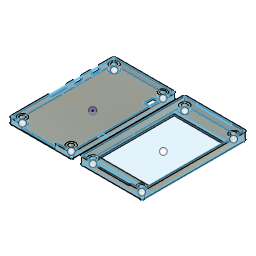
ProjectSpectre (Autodesk Fusion 360 design; units mm, degrees)
Autodesk Fusion 360 part; units mm, degrees
sketch "Sketch1" plane through (0, 0, 0) normal (0, 0, 1) x (1, 0, 0)
  line L0 (-25.25, 0) -> (-25.25, 43.25)
  line L1 (25.25, 0) -> (25.25, 43.25)
  line L2 (-25.25, 0) -> (-25.25, -43.25)
  line L3 (25.25, 0) -> (25.25, -43.25)
  line L4 (-25.25, 43.25) -> (25.25, 43.25)
  line L5 (-25.25, -43.25) -> (25.25, -43.25)
  circle A0 centre (-20.75, 39) radius 2.1
  circle A1 centre (20.75, 39) radius 2.1
  circle A2 centre (-20.75, -39) radius 2.1
  circle A3 centre (20.75, -39) radius 2.1
  line L6 (-25.25, 43.25, 0) -> (-25.25, 43.25, 4.5)
  line L7 (25.25, 43.25, 0) -> (25.25, 43.25, 4.5)
  line L8 (25.25, -43.25, 0) -> (25.25, -43.25, 4.5)
  line L9 (-25.25, -43.25, 0) -> (-25.25, -43.25, 4.5)
  line L10 (25.25, 43.25, 4.5) -> (25.25, -43.25, 4.5)
  line L11 (-25.25, -43.25, 4.5) -> (-25.25, 43.25, 4.5)
  line L12 (-25.25, 43.25, 4.5) -> (25.25, 43.25, 4.5)
  line L13 (-25.25, 43.25, 4.5) -> (-25.25, 31.55, 4.5)
  line L14 (-25.25, 31.55, 4.5) -> (-25.25, 31.55, 1)
  line L15 (-25.25, 31.55, 1) -> (-25.25, 24.55, 1)
  line L16 (-25.25, 24.55, 1) -> (-25.25, 24.55, 4.5)
  line L17 (-25.25, 24.55, 4.5) -> (-25.25, 16.65, 4.5)
  line L18 (-25.25, 16.65, 4.5) -> (-25.25, 16.65, 1)
  line L19 (-25.25, 16.65, 1) -> (-25.25, 9.65, 1)
  line L20 (-25.25, 9.65, 1) -> (-25.25, 9.65, 4.5)
  line L21 (21.95, 35.45) -> (21.95, 27.45)
  line L22 (21.95, 27.45) -> (15.85, 27.45)
  line L23 (15.85, 27.45) -> (15.85, 35.45)
  line L24 (15.85, 35.45) -> (21.95, 35.45)
  line L25 (-25.25, 9.65, 4.5) -> (-25.25, 4, 4.5)
  line L26 (-25.25, 4, 4.5) -> (-25.25, 4, 2.5)
  line L27 (-25.25, 4, 2.5) -> (-25.25, -11, 2.5)
  line L28 (-25.25, -11, 2.5) -> (-25.25, -11, 4.5)
  line L29 (24.25, -16.75) -> (24.25, -12.45)
  line L30 (24.25, -12.45) -> (21.35, -12.45)
  line L31 (21.35, -12.45) -> (21.35, -16.75)
  line L32 (21.35, -16.75) -> (24.25, -16.75)
  circle A4 centre (20.75, -39) radius 3.75
  circle A5 centre (-20.75, -39) radius 3.75
  circle A6 centre (-20.75, 39) radius 3.75
  circle A7 centre (20.75, 39) radius 3.5
  line L33 (-25.25, -43.25, 4.5) -> (-15.75, -43.25, 4.5)
  line L34 (-15.75, -43.25, 4.5) -> (-15.75, -43.25, 1)
  line L35 (-15.75, -43.25, 1) -> (13.05, -43.25, 1)
  line L36 (13.05, -43.25, 1) -> (13.05, -43.25, 4.5)
  line L37 (13.05, -43.25, 4.5) -> (25.25, -43.25, 4.5)
  line L38 (24.25, -12.45) -> (21.35, -12.45)
  line L39 (21.95, 27.45) -> (15.85, 27.45)
  line L40 (-25.25, -43.25, 0) -> (-25.25, -43.25, 4.5)
  line L41 (-25.25, 4, 4.5) -> (-25.25, 4, 2.5)
  line L42 (-25.25, 0) -> (-25.25, -43.25)
  line L43 (-25.25, -43.25, 4.5) -> (-15.75, -43.25, 4.5)
  line L44 (-25.25, 4, 2.5) -> (-25.25, -11, 2.5)
  circle A8 centre (20.75, 39) radius 2.1
  line L45 (-25.25, -43.25) -> (25.25, -43.25)
  line L46 (-25.25, 31.55, 4.5) -> (-25.25, 31.55, 1)
  line L47 (25.25, -43.25, 0) -> (25.25, -43.25, 4.5)
  circle A9 centre (20.75, -39) radius 3.75
  line L48 (15.85, 27.45) -> (15.85, 35.45)
  line L49 (-25.25, 0) -> (-25.25, 43.25)
  line L50 (21.35, -16.75) -> (24.25, -16.75)
  line L51 (-25.25, 43.25, 0) -> (-25.25, 43.25, 4.5)
  line L52 (13.05, -43.25, 4.5) -> (25.25, -43.25, 4.5)
  circle A10 centre (-20.75, 39) radius 2.1
  line L53 (21.35, -12.45) -> (21.35, -16.75)
  circle A11 centre (20.75, 39) radius 3.5
  line L54 (15.85, 35.45) -> (21.95, 35.45)
  line L55 (25.25, 0) -> (25.25, -43.25)
  line L56 (24.25, -16.75) -> (24.25, -12.45)
  line L57 (13.05, -43.25, 1) -> (13.05, -43.25, 4.5)
  circle A12 centre (20.75, -39) radius 2.1
  line L58 (-25.25, 43.25) -> (25.25, 43.25)
  line L59 (21.95, 35.45) -> (21.95, 27.45)
  line L60 (-25.25, 43.25, 4.5) -> (25.25, 43.25, 4.5)
  line L61 (25.25, 43.25, 0) -> (25.25, 43.25, 4.5)
  circle A13 centre (-20.75, 39) radius 3.75
  line L62 (-25.25, -43.25, 4.5) -> (-25.25, 43.25, 4.5)
  line L63 (-25.25, 9.65, 4.5) -> (-25.25, 4, 4.5)
  line L64 (25.25, 0) -> (25.25, 43.25)
  line L65 (25.25, 43.25, 4.5) -> (25.25, -43.25, 4.5)
  line L66 (-25.25, 43.25, 4.5) -> (-25.25, 31.55, 4.5)
  line L67 (-25.25, 31.55, 1) -> (-25.25, 24.55, 1)
  line L68 (-15.75, -43.25, 1) -> (13.05, -43.25, 1)
  line L69 (-25.25, 24.55, 1) -> (-25.25, 24.55, 4.5)
  line L70 (-25.25, 16.65, 4.5) -> (-25.25, 16.65, 1)
  line L71 (-25.25, 16.65, 1) -> (-25.25, 9.65, 1)
  line L72 (-15.75, -43.25, 4.5) -> (-15.75, -43.25, 1)
  line L73 (-25.25, 9.65, 1) -> (-25.25, 9.65, 4.5)
  line L74 (-25.25, -11, 2.5) -> (-25.25, -11, 4.5)
  circle A14 centre (-20.75, -39) radius 3.75
  line L75 (-25.25, 24.55, 4.5) -> (-25.25, 16.65, 4.5)
  circle A15 centre (-20.75, -39) radius 2.1
  dimension "d5" = 41.5
  dimension "d7" = 78
  dimension "d8" = 25.25
  dimension "d9" = 25.25
  dimension "d12" = 43.25
  dimension "d13" = 43.25
  dimension "d14" = 43.25
  dimension "d15" = 43.25
  dimension "d16" = 4.2
  dimension "d17" = 4.2
  dimension "d18" = 4.2
  dimension "d19" = 4.2
  dimension "d28" = 4.5
  dimension "d29" = 4.5
  dimension "d30" = 4.5
  dimension "d31" = 4.5
  dimension "d32" = 11.7
  dimension "d33" = 3.5
  dimension "d34" = 7
  dimension "d35" = 3.5
  dimension "d36" = 7.9
  dimension "d37" = 3.5
  dimension "d38" = 7
  dimension "d39" = 3.5
  dimension "d42" = 8
  dimension "d43" = 6.1
  dimension "d44" = 8
  dimension "d45" = 5.65
  dimension "d46" = 2
  dimension "d47" = 15
  dimension "d54" = 4.3
  dimension "d55" = 2.9
  dimension "d56" = 4.3
  dimension "d57" = 7.5
  dimension "d58" = 7.5
  dimension "d59" = 7.5
  dimension "d60" = 7
  dimension "d62" = 9.5
  dimension "d63" = 3.5
  dimension "d64" = 28.8
  dimension "d65" = 3.5
  dimension "d100" = 41.5
  dimension "d101" = 78
  dimension "d103" = 43.25
  dimension "d104" = 43.25
  dimension "d105" = 43.25
  dimension "d106" = 43.25
  dimension "d107" = 4.2
  dimension "d108" = 4.2
  dimension "d109" = 4.2
  dimension "d110" = 4.2
  dimension "d111" = 4.5
  dimension "d112" = 4.5
  dimension "d113" = 4.5
  dimension "d114" = 4.5
  dimension "d115" = 11.7
  dimension "d116" = 3.5
  dimension "d117" = 7
  dimension "d118" = 3.5
  dimension "d119" = 7.9
  dimension "d120" = 3.5
  dimension "d121" = 7
  dimension "d122" = 3.5
  dimension "d123" = 8
  dimension "d124" = 6.1
  dimension "d125" = 8
  dimension "d126" = 5.65
  dimension "d127" = 2
  dimension "d128" = 15
  dimension "d129" = 4.3
  dimension "d130" = 2.9
  dimension "d131" = 4.3
  dimension "d132" = 7.5
  dimension "d133" = 7.5
  dimension "d134" = 7.5
  dimension "d135" = 7
  dimension "d136" = 9.5
  dimension "d137" = 3.5
  dimension "d138" = 28.8
  dimension "d139" = 3.5
  constraint perpendicular L22 L23
  constraint perpendicular L29 L30
  constraint perpendicular L30 L31
  constraint concentric A3 A4
  constraint concentric A2 A5
  constraint concentric A0 A6
  constraint concentric A1 A7
  constraint perpendicular L39 L48
  constraint perpendicular L38 L56
  constraint perpendicular L38 L53
  constraint concentric A9 A12
  constraint concentric A14 A15
  constraint concentric A10 A13
  constraint concentric A8 A11
  measures "d5" distance of A0.centre A1.centre
  measures "d7" distance of A0.centre A2.centre
  measures "d8" distance of origin L1.start
  measures "d9" distance of origin L0.start
  measures "d12" distance of L0.start L0.end
  measures "d13" distance of L1.start L1.end
  measures "d14" distance of L0.start L2.end
  measures "d15" distance of L1.start L3.end
  measures "d16" diameter of A0
  measures "d17" diameter of A1
  measures "d18" diameter of A2
  measures "d19" diameter of A3
  measures "d28" distance of L0.end L4.start
  measures "d29" distance of L1.end L4.end
  measures "d30" distance of L3.end L5.end
  measures "d31" distance of L2.end L5.start
  measures "d42" distance of L21.start L21.end
  measures "d43" distance of L21.end L22.end
  measures "d44" distance of L22.end L23.end
  measures "d54" distance of L29.start L29.end
  measures "d55" distance of L29.end L30.end
  measures "d56" distance of L30.end L31.end
  measures "d57" diameter of A4
  measures "d58" diameter of A5
  measures "d59" diameter of A6
  measures "d60" diameter of A7
  measures "d100" distance of A1.centre A0.centre
  measures "d101" distance of A2.centre A0.centre
  measures "d103" distance of L0.start L0.end
  measures "d104" distance of L1.end L1.start
  measures "d105" distance of L0.start L2.end
  measures "d106" distance of L3.end L1.start
  measures "d107" diameter of A10
  measures "d108" diameter of A8
  measures "d109" diameter of A15
  measures "d110" diameter of A12
  measures "d111" distance of L0.end L4.start
  measures "d112" distance of L1.end L4.end
  measures "d113" distance of L3.end L5.end
  measures "d114" distance of L2.end L5.start
  measures "d123" distance of L21.start L21.end
  measures "d124" distance of L22.end L21.end
  measures "d125" distance of L22.end L23.end
  measures "d129" distance of L29.start L29.end
  measures "d130" distance of L30.end L29.end
  measures "d131" distance of L31.end L30.end
  measures "d132" diameter of A9
  measures "d133" diameter of A14
  measures "d134" diameter of A13
  measures "d135" diameter of A11
extrude "Extrude1" add sketch "Sketch1" against normal blind 1.5 contours L1 L3 L7 L8 L10 L47 L55 L61 L64 L65 in plane through (25.25, 0, 0) normal (1, 0, 0) makes body 1
extrude "Extrude2" add sketch "Sketch1" along normal blind 1.5 contours L4 L6 L7 L12 L51 L58 L60 L61 in plane through (0, 43.25, 0) normal (0, 1, 0) bodies 1
extrude "Extrude3" add 1 faces at (-25.25, 43.75, 1.5) along direction (-1, 0, 0) blind 1.5 on bodies 1 bodies 1
extrude "Extrude4" add sketch "Sketch1" against normal blind 1.5 contours L0 L2 L6 L9 L11 L13 L14 L15 L16 L17 L18 L19 L20 L25 L26 L27 L28 L40 L41 L42 L44 L46 L49 L51 L62 L63 L66 L67 L69 L70 L71 L73 L74 L75 in plane through (-25.25, 0, 0) normal (1, 0, 0) bodies 1
extrude "Extrude5" cut 1 faces at (23.75, 14.4167, 1.5) along direction (1, 0, 0) blind 3 on bodies 1 bodies 1
extrude "Extrude6" add 1 faces at (25.25, 44.25, 1.5) along direction (1, 0, 0) blind 1.5 on bodies 1 bodies 1
extrude "Extrude7" add sketch "Sketch1" against normal blind 1.5 contours L1 L3 L7 L8 L10 L47 L55 L61 L64 L65 in plane through (25.25, 0, 0) normal (1, 0, 0) bodies 1
extrude "Extrude8" add sketch "Sketch1" against normal blind 1.5 contours L1 L3 L7 L8 L10 L47 L55 L61 L64 L65 in plane through (25.25, 0, 0) normal (1, 0, 0) bodies 1
extrude "Extrude9" add 1 faces at (25.75, 43.25, 3) along direction (0, -1, 0) blind 86.5 on bodies 1 bodies 1
extrude "Extrude10" cut 1 faces at (23.75, 14.4167, 1.5) along direction (1, 0, 0) blind 1.5 on bodies 1 bodies 1
extrude "Extrude11" add sketch "Sketch1" against normal blind 1.5 separate body contours L5 L8 L9 L33 L34 L35 L36 L37 L40 L43 L45 L47 L52 L57 L68 L72 in plane through (0, -43.25, 0) normal (0, 1, 0) makes body 2
extrude "Extrude12" add 2 faces at (-25.75, -43.25, 1.5) (25.75, -43.25, 3) along direction (0, -1, 0) blind 1.5 on bodies 1 bodies 1 2
extrude "Extrude13" add sketch "Sketch1" against normal blind 1.5 separate body contours L0 L1 L2 L3 L4 L5 L42 L45 L49 L55 L58 L64 | A0 A10 | A1 A8 | A2 A15 | A3 A12 | A4 A9 | A5 A14 | A6 A13 | A7 A11 makes body 3
extrude "Extrude14" add 1 faces at (26.25, -14.4167, 0) along direction (0, 0, -1) blind 1.5 on bodies 1 bodies 1 3
extrude "Extrude15" add sketch "Sketch1" along normal blind 4.5 contours A4 A9 | A5 A14 | A6 A13 | A7 A11 bodies 1
fillet "Fillet1" radius 1.5 4 edges at (0, 44.75, -1.5) (26.75, 0, -1.5) (-26.75, 0, -1.5) (0, -44.75, -1.5) on bodies 1
fillet "Fillet2" radius 2 8 edges at (-26.75, 44.75, 2.25) (-26.3107, 44.3107, -1.0607) (26.75, 44.75, 2.25) (26.3107, 44.3107, -1.0607) (26.75, -44.75, 2.25) (26.3107, -44.3107, -1.0607) (-26.3107, -44.3107, -1.0607) (-26.75, -44.75, 2.25) on bodies 1
sketch "Sketch2" plane through (0, 0, 0) normal (0, 0, 1) x (1, 0, 0)
  circle A0 centre (80.75, -39) radius 3.75
  line L0 (34.75, -43.25) -> (85.25, -43.25)
  circle A1 centre (80.75, -39) radius 3.75
  circle A2 centre (39.25, -39) radius 2.1
  line L1 (85.25, 0) -> (85.25, 43.25)
  line L2 (85.25, 0) -> (85.25, -43.25)
  line L3 (85.25, 0) -> (85.25, -43.25)
  circle A3 centre (80.75, -39) radius 2.1
  line L4 (34.75, 0) -> (34.75, -43.25)
  line L5 (85.25, 0) -> (85.25, 43.25)
  line L6 (34.75, 43.25) -> (85.25, 43.25)
  circle A4 centre (39.25, -39) radius 3.75
  line L7 (34.75, 0) -> (34.75, -43.25)
  circle A5 centre (39.25, -39) radius 3.75
  line L8 (34.75, 43.25) -> (85.25, 43.25)
  circle A6 centre (80.75, -39) radius 2.1
  line L9 (34.75, 0) -> (34.75, 43.25)
  line L10 (34.75, 0) -> (34.75, 43.25)
  circle A7 centre (39.25, 39) radius 3.75
  circle A8 centre (39.25, 39) radius 2.1
  circle A9 centre (39.25, 39) radius 2.1
  circle A10 centre (80.75, 39) radius 2.1
  circle A11 centre (80.75, 39) radius 3.5
  circle A12 centre (39.25, -39) radius 2.1
  circle A13 centre (80.75, 39) radius 3.5
  line L11 (34.75, -43.25) -> (85.25, -43.25)
  circle A14 centre (80.75, 39) radius 2.1
  circle A15 centre (39.25, 39) radius 3.75
  line L12 (85.25, 43.25, 0) -> (85.25, 43.25, 6.1)
  line L13 (34.75, 43.25, 0) -> (34.75, 43.25, 6.1)
  line L14 (34.75, -43.25, 0) -> (34.75, -43.25, 6.1)
  line L15 (85.25, -43.25, 0) -> (85.25, -43.25, 6.1)
  line L16 (34.75, 43.25, 6.1) -> (34.75, -43.25, 6.1)
  line L17 (85.25, -43.25, 6.1) -> (34.75, -43.25, 6.1)
  line L18 (85.25, -43.25, 6.1) -> (85.25, 43.25, 6.1)
  line L19 (85.25, 43.25, 6.1) -> (34.75, 43.25, 6.1)
  line L20 (60, -34.75) -> (85.25, -34.75)
  line L21 (60, -34.75) -> (34.75, -34.75)
  line L22 (58.3127, 33.95) -> (34.75, 33.95)
  line L23 (58.3127, 33.95) -> (85.25, 33.95)
  line L24 (34.75, 43.25, 0) -> (34.75, 43.25, -1.5)
  line L25 (85.25, 43.25, 0) -> (85.25, 43.25, -1.5)
  line L26 (34.75, -43.25, 0) -> (34.75, -43.25, -1.5)
  line L27 (85.25, -43.25, 0) -> (85.25, -43.25, -1.5)
  line L28 (85.25, -43.25, -1.5) -> (85.25, 43.25, -1.5)
  line L29 (34.75, 43.25, -1.5) -> (34.75, -43.25, -1.5)
  line L30 (34.75, 43.25, 6.1) -> (45.55, 43.25, 6.1)
  line L31 (45.55, 43.25, 6.1) -> (45.55, 43.25, 5.1)
  line L32 (45.55, 43.25, 5.1) -> (74.55, 43.25, 5.1)
  line L33 (74.55, 43.25, 5.1) -> (74.55, 43.25, 6.1)
  line L34 (74.55, 43.25, 6.1) -> (45.55, 43.25, 6.1)
  point P0 (60, 0)
  dimension "d140" = 41.5
  dimension "d141" = 78
  dimension "d142" = 25.25
  dimension "d143" = 25.25
  dimension "d144" = 43.25
  dimension "d145" = 43.25
  dimension "d146" = 43.25
  dimension "d147" = 43.25
  dimension "d148" = 4.2
  dimension "d149" = 4.2
  dimension "d150" = 4.2
  dimension "d151" = 4.2
  dimension "d173" = 7.5
  dimension "d174" = 7.5
  dimension "d175" = 7.5
  dimension "d176" = 7
  dimension "d181" = 41.5
  dimension "d182" = 78
  dimension "d183" = 43.25
  dimension "d184" = 43.25
  dimension "d185" = 43.25
  dimension "d186" = 43.25
  dimension "d187" = 4.2
  dimension "d188" = 4.2
  dimension "d189" = 4.2
  dimension "d190" = 4.2
  dimension "d212" = 7.5
  dimension "d213" = 7.5
  dimension "d214" = 7.5
  dimension "d215" = 7
  dimension "d220" = 6.1
  dimension "d221" = 6.1
  dimension "d222" = 6.1
  dimension "d223" = 6.1
  dimension "d273" = 1.5
  dimension "d274" = 1.5
  dimension "d275" = 1.5
  dimension "d276" = 1.5
  dimension "d289" = 10.8
  dimension "d290" = 1
  dimension "d291" = 29
  constraint concentric A1 A6
  constraint concentric A2 A5
  constraint concentric A7 A9
  constraint concentric A11 A14
  constraint concentric A0 A3
  constraint concentric A4 A12
  constraint concentric A8 A15
  constraint concentric A10 A13
  constraint coincident L2 L20.end
  constraint perpendicular L2 L20
  constraint coincident L7 L21.end
  constraint perpendicular L7 L21
  constraint coincident L10 L22.end
  constraint perpendicular L10 L22
  constraint coincident L5 L23.end
  constraint perpendicular L5 L23
  measures "d140" distance of A10.centre A7.centre
  measures "d141" distance of A2.centre A7.centre
  measures "d142" distance of P0 L1.start
  measures "d143" distance of L4.start P0
  measures "d144" distance of L4.start L6.start
  measures "d145" distance of L1.end L1.start
  measures "d146" distance of L4.start L0.start
  measures "d147" distance of L0.end L1.start
  measures "d148" diameter of A9
  measures "d149" diameter of A14
  measures "d150" diameter of A2
  measures "d151" diameter of A6
  measures "d173" diameter of A1
  measures "d174" diameter of A5
  measures "d175" diameter of A7
  measures "d176" diameter of A11
  measures "d181" distance of A7.centre A10.centre
  measures "d182" distance of A2.centre A7.centre
  measures "d183" distance of L4.start L6.start
  measures "d184" distance of L1.end L1.start
  measures "d185" distance of L0.start L4.start
  measures "d186" distance of L0.end L1.start
  measures "d187" diameter of A8
  measures "d188" diameter of A10
  measures "d189" diameter of A12
  measures "d190" diameter of A3
  measures "d212" diameter of A0
  measures "d213" diameter of A4
  measures "d214" diameter of A15
  measures "d215" diameter of A13
  measures "d220" distance of L1.end L5.end
  measures "d221" distance of L6.start L8.start
  measures "d222" distance of L0.start L4.end
  measures "d223" distance of L0.end L2.end
  measures "d273" distance of L6.start L8.start
  measures "d274" distance of L1.end L5.end
  measures "d275" distance of L0.start L4.end
  measures "d276" distance of L0.end L2.end
extrude "Extrude16" add sketch "Sketch2" against normal blind 1.5 separate body contours L0 L11 L14 L15 L17 in plane through (0, -43.25, 0) normal (0, 1, 0) makes body 4
extrude "Extrude17" add sketch "Sketch2" along normal blind 1.5 separate body contours L1 L2 L3 L5 L12 L15 L18 in plane through (85.25, 0, 0) normal (1, 0, 0) makes body 5
extrude "Extrude18" add sketch "Sketch2" along normal blind 1.5 separate body contours L6 L8 L12 L13 L19 L30 L31 L32 L33 | L19 L31 L32 L33 L34 in plane through (0, 43.25, 0) normal (0, 1, 0) makes body 6
extrude "Extrude19" add 1 faces at (34.75, 43.75, 2.0333) along direction (-1, 0, 0) blind 1.5 on bodies 6 bodies 6
extrude "Extrude20" add 1 faces at (34.75, -43.75, 2.0333) along direction (-1, 0, 0) blind 1.5 on bodies 4 bodies 4
extrude "Extrude21" add sketch "Sketch2" along normal blind 1.5 contours L4 L7 L9 L10 L13 L14 L16 in plane through (34.75, 0, 0) normal (1, 0, 0) bodies 4 6
extrude "Extrude22" add sketch "Sketch2" along normal blind 1.5 contours L4 L7 L9 L10 L13 L14 L16 in plane through (34.75, 0, 0) normal (1, 0, 0) bodies 4
extrude "Extrude23" add 1 faces at (34.25, 43.25, 4.0667) along direction (0, -1, 0) blind 87 on bodies 4 bodies 4
extrude "Extrude24" cut 1 faces at (36.25, -14.4167, 2.0333) along direction (-1, 0, 0) blind 1.5 on bodies 4 bodies 4
extrude "Extrude25" add sketch "Sketch2" against normal blind 1.5 separate body contours A0 A1 | L0 L2 L3 L4 L7 L11 L20 L21 | L1 L5 L6 L8 L9 L10 L22 L23 | A2 A12 | A3 A6 | A4 A5 | A7 A15 | A8 A9 | A10 A14 | A11 A13 makes body 7 at (51.5833, -37.5833, 0) makes body 8 at (68.4167, 37.05, 0)
extrude "Extrude26" add 1 faces at (85.25, -43.75, 2.0333) along direction (1, 0, 0) blind 1.5 on bodies 4 bodies 4 8 5 7
extrude "Extrude27" add 1 faces at (85.25, 44.25, 4.0667) along direction (1, 0, 0) blind 1.5 on bodies 4 bodies 4 8
extrude "Extrude28" add 1 faces at (86.25, 11.3167, 0) along direction (0, 0, -1) blind 1.5 on bodies 4 bodies 4
extrude "Extrude29" add sketch "Sketch2" along normal blind 4.9 separate body contours A0 A1 | A4 A5 | A7 A15 | A11 A13 makes body 9 at (78.4341, 36.3758, 3.2667) makes body 10 at (42.9814, 38.6266, 3.2667) makes body 11 at (84.4814, -39.3734, 3.2667) makes body 12 at (42.9814, -39.3734, 3.2667)
fillet "Fillet3" radius 1.5 4 edges at (60, -44.75, -1.5) (86.75, 0, -1.5) (60, 44.75, -1.5) (33.25, 0, -1.5) on bodies 4
fillet "Fillet4" radius 2 6 edges at (33.25, -44.75, 3.05) (33.6893, -44.3107, -1.0607) (86.75, -44.75, 3.05) (86.3107, -44.3107, -1.0607) (33.6893, 44.3107, -1.0607) (33.25, 44.75, 3.05) on bodies 4
hole "Hole1" at (80.75, -39, 0) at (39.25, -39, 0) at (80.75, 39, 0) at (39.25, 39, 0) direction (0, 0, -1) diameter 3 depth 35 tip angle 118 bodies 4
extrude "Extrude30" add 4 faces at (42.4282, -39.2906, 4.9) (83.936, -39.1863, 4.9) (42.4282, 38.7094, 4.9) (83.7625, 38.7218, 4.9) along direction (0, 0, -1) blind 5.5 on bodies 9 10 11 12 bodies 4 12 9 10 11
extrude "Extrude34" add 1 faces at (51.5833, -34.75, -0.5) along direction (0, 1, 0) blind 3.5 on bodies 4 bodies 4
extrude "Extrude35" add 1 faces at (68.4167, 33.95, -0.5) along direction (0, -1, 0) blind 1.5 on bodies 4 bodies 4
extrude "Extrude36" add sketch "Sketch2" along normal blind 2 contours L4 L7 L9 L10 L24 L26 L29 in plane through (34.75, 0, 0) normal (1, 0, 0) bodies 4
extrude "Extrude37" add sketch "Sketch2" against normal blind 2 contours L1 L2 L3 L5 L25 L27 L28 in plane through (85.25, 0, 0) normal (1, 0, 0) bodies 4
extrude "Extrude38" cut 4 faces at (42.4282, 38.7094, 4.9) (83.7625, 38.7218, 4.9) (42.4282, -39.2906, 4.9) (83.936, -39.1863, 4.9) along direction (0, 0, -1) blind 0.8 on bodies 4 bodies 4
fillet "Fillet6" radius 2 2 edges at (86.75, 44.75, 3.05) (86.3107, 44.3107, -1.0607) on bodies 4
extrude "Extrude39" cut sketch "Sketch2" along normal blind 1.5 contours L19 L31 L32 L33 L34 in plane through (0, 43.25, 0) normal (0, 1, 0) bodies 4
extrude "Extrude40" cut 1 faces at (45.55, 43.75, 5.7667) along direction (-1, 0, 0) blind 1.3 on bodies 4 bodies 4
extrude "Extrude41" add 1 faces at (74.55, 43.75, 5.4333) along direction (-1, 0, 0) blind 1.3 on bodies 4 bodies 4
extrude "Extrude42" cut sketch "Sketch2" against normal blind 140 contours L19 L31 L32 L33 L34 in plane through (0, 43.25, 0) normal (0, 1, 0) bodies 4
extrude "Extrude43" add 1 faces at (45.55, -43.75, 5.7667) along direction (1, 0, 0) blind 1.3 on bodies 4 bodies 4
extrude "Extrude44" cut 1 faces at (46.85, -43.75, 5.7667) along direction (-1, 0, 0) blind 2.6 on bodies 4 bodies 4
extrude "Extrude45" add 1 faces at (74.55, -43.75, 5.4333) along direction (-1, 0, 0) blind 1.3 on bodies 4 bodies 4
extrude "Extrude46" add 1 faces at (73.25, 43.75, 5.4333) along direction (-1, 0, 0) blind 29 on bodies 4 bodies 4
extrude "Extrude47" add 1 faces at (44.25, -43.75, 5.7667) along direction (1, 0, 0) blind 2.6 on bodies 4 bodies 4
extrude "Extrude48" cut 1 faces at (73.25, -43.75, 5.4333) along direction (1, 0, 0) blind 2.6 on bodies 4 bodies 4
